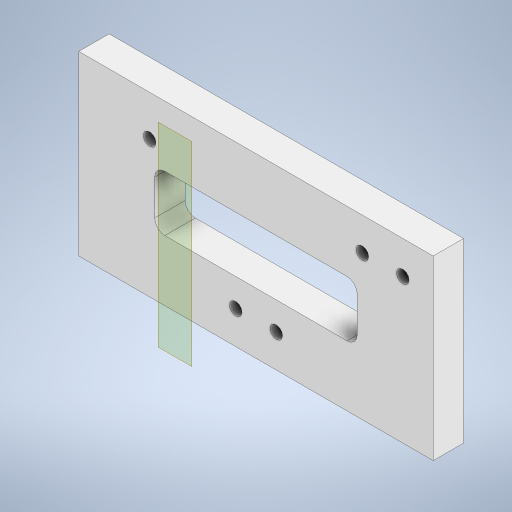
# Autodesk Inventor part: 61_CPY
Saved by Autodesk Inventor 2024.3 (Build 283343000, 343)
## iProperties
Created: 2024-09-08
Part Number: 61_CPY
Material: 아크릴, 선명
Document SubType Name: Modeling
Designer: 구지현
Density: 1.19 g/cm^3
Appearance: 흰색
Author: 구지현
Autodesk Inventor part; units mm, degrees
ref_plane "YZ Plane" through (0, 0, 0) normal (1, 0, 0) x (0, 1, 0)
ref_plane "XZ Plane" through (0, 0, 0) normal (0, 1, 0) x (-1, 0, 0)
ref_plane "XY Plane" through (0, 0, 0) normal (0, 0, 1) x (1, 0, 0)
ref_plane "작업 평면1" through (28, 0, 12) normal (0, 0, -1) x (-1, 0, 0)
sketch "스케치1" plane through (0, 0, 0) normal (0, 0, 1) x (1, 0, 0)
  line L0 (0, 0) -> (6, 0) projected
  line L1 (6, 0) -> (6, 35) projected
  line L2 (0, 35) -> (6, 35) projected
  line L3 (0, 0) -> (0, 35) projected
  line L4 (0, 35) -> (70, 35)
  line L5 (70, 35) -> (70, 0)
  line L6 (70, 0) -> (0, 0)
  line L7 (0, 0) -> (0, 35)
  dimension "d0" = 70
  constraints: 8 end point, 2 parallel, 1 horizontal, 1 perpendicular
  measures "d0" distance of L5.end L6.end
extrude "돌출1" add sketch "스케치1" along normal blind 6
sketch "스케치2" plane through (0, 0, 6) normal (0, 0, 1) x (1, 0, 0)
  circle A0 centre (39, 6.5) radius 1.25 projected
  circle A1 centre (31, 6.5) radius 1.25 projected
  line L0 (25, 3) -> (45, 3) projected
  line L1 (45, 3) -> (45, 10) projected
  line L2 (45, 10) -> (25, 10) projected
  line L3 (25, 10) -> (25, 3) projected
  point P0 (0, 0)
extrude "돌출2" cut sketch "스케치2" against normal blind 6 contours A0 | A1
sketch "스케치3" plane through (0, 0, 6) normal (0, 0, 1) x (1, 0, 0)
  circle A0 centre (56, 28.5) radius 1.25 projected
  circle A1 centre (64, 28.5) radius 1.25 projected
  circle A2 centre (56, 28.5) radius 1.25 projected
  line L0 (50, 32) -> (70, 32) projected
  line L1 (70, 32) -> (70, 25) projected
  line L2 (70, 25) -> (50, 25) projected
  line L3 (50, 25) -> (50, 32) projected
  circle A3 centre (12.5, 27) radius 1.25 projected
  line L4 (9, 32) -> (16, 32) projected
  line L5 (16, 22) -> (16, 32) projected
  line L6 (9, 22) -> (16, 22) projected
  line L7 (9, 32) -> (9, 22) projected
  circle A4 centre (14, 27) radius 1.25 projected
  line L8 (19, 22) -> (19, 32) projected
  line L9 (19, 32) -> (9, 32) projected
  line L10 (9, 32) -> (9, 22) projected
  line L11 (9, 22) -> (19, 22) projected
  point P0 (0, 0)
extrude "돌출3" cut sketch "스케치3" against normal blind 6 contours A0 | A1 | A3 A4 | A3 A4 picked at (13.4055, 26.9043) picked at (14.7375, 27.1015)
sketch "스케치4" plane through (0, 0, 0) normal (0, 0, -1) x (-1, 0, 0)
  line L0 (0, 35) -> (0, 0) projected
  line L1 (-70, 0) -> (-70, 35) projected
  line L2 (-70, 35) -> (0, 35) projected
  line L3 (0, 0) -> (-70, 0) projected
  line L4 (-55, 23) -> (-15, 23)
  line L5 (-15, 23) -> (-15, 12)
  line L6 (-15, 12) -> (-55, 12)
  line L7 (-55, 12) -> (-55, 23)
  point P0 (-55, 18.9013)
  point P1 (-37.9373, 23)
  point P2 (-15, 18.9013)
  point P3 (-36.2312, 12)
  dimension "d7" = 15
  dimension "d8" = 15
  dimension "d9" = 12
  dimension "d10" = 12
  constraints: 8 end point, 2 parallel, 1 horizontal, 1 perpendicular
  measures "d7" distance from line of L0 point (-15, 18.901)
  measures "d8" distance from line of L1 point (-55, 18.901)
  measures "d9" distance from line of L2 point (-37.937, 23)
  measures "d10" distance from line of L3 point (-36.231, 12)
extrude "돌출4" cut sketch "스케치4" against normal blind 6 contours L4 L5 L6 L7
fillet "모깎기1" radius 2 4 edges at (55, 23, 3) (15, 23, 3) (15, 12, 3) (55, 12, 3)
